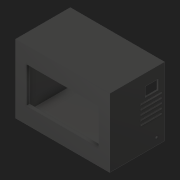
# Autodesk Inventor part: GA06
Saved by Autodesk Inventor 2017 (Build 210142000, 142)
## iProperties
Created: 2018-11-17
Part Number: GA06
Material: ABS Plastic
Document SubType Name: Modeling
Designer: Dell
Density: 1.06 g/cm^3
Appearance: Smooth - Black
Author: Dell
Autodesk Inventor part; units mm, degrees
ref_plane "YZ Plane" through (0, 0, 0) normal (1, 0, 0) x (0, 1, 0)
ref_plane "XZ Plane" through (0, 0, 0) normal (0, 1, 0) x (-1, 0, 0)
ref_plane "XY Plane" through (0, 0, 0) normal (0, 0, 1) x (1, 0, 0)
sketch "Sketch1" plane through (0, 0, 0) normal (0, 0, 1) x (1, 0, 0)
  line L0 (0, 0) -> (0, 70) construction
  circle A0 centre (0, 0) radius 2.5
  circle A1 centre (0, 70) radius 2.5
  line L1 (0, 0) -> (125, 0) construction
  circle A2 centre (125, 0) radius 2.5
  circle A3 centre (125, 70) radius 2.5
  line L2 (-8.5, -16) -> (133.5, -16)
  line L3 (133.5, -16) -> (133.5, 86)
  line L4 (133.5, 86) -> (-8.5, 86)
  line L5 (-8.5, 86) -> (-8.5, -16)
  point P0 (62.5, 0)
  point P1 (62.5, -16)
  point P2 (0, 35)
  point P3 (-8.5, 35)
  dimension "d0" = 70
  dimension "d1" = 5
  dimension "d2" = 5
  dimension "d3" = 5
  dimension "d4" = 5
  dimension "d5" = 125
  dimension "d6" = 142
  dimension "d7" = 102
  constraints: 12 end point, 4 centre point, 4 midpoint, 3 coincident, 2 horizontal, 2 horizontal alignment, 2 parallel, 2 vertical alignment, 1 perpendicular, 1 vertical
  measures "d0" distance of L0.start L0.end
  measures "d1" diameter of A0
  measures "d2" diameter of A1
  measures "d3" diameter of A2
  measures "d4" diameter of A3
  measures "d5" distance of L1.start L1.end
  measures "d6" distance of L4.end L3.end
  measures "d7" distance of L3.end L2.end
extrude "Extrusion1" add sketch "Sketch1" along normal blind 5
sketch "Sketch2" plane through (0, 0, 5) normal (0, 0, 1) x (1, 0, 0)
  line L0 (6.5, 60) -> (118.5, 60)
  line L1 (118.5, 60) -> (118.5, 10)
  line L2 (118.5, 10) -> (6.5, 10)
  line L3 (6.5, 10) -> (6.5, 60)
  line L4 (-8.5, 86) -> (-8.5, -16) projected
  line L5 (133.5, 86) -> (-8.5, 86) projected
  point P0 (0, 0)
  point P1 (62.5, 60)
  point P2 (62.5, 86)
  point P3 (6.5, 35)
  point P4 (-8.5, 35)
  dimension "d10" = 15
  dimension "d11" = 50
  constraints: 8 end point, 4 midpoint, 2 parallel, 1 horizontal, 1 horizontal alignment, 1 perpendicular, 1 vertical alignment
  measures "d10" distance between parallel lines of L4 L3
  measures "d11" distance of L0.end L1.end
extrude "Extrusion2" cut sketch "Sketch2" against normal through all
sketch "Sketch3" plane through (-8.5, 86, 0) normal (0, 1, 0) x (1, 0, 0)
  line L0 (142, 0) -> (142, -5) projected
  line L1 (142, -5) -> (0, -5)
  line L2 (0, -5) -> (0, 80)
  line L3 (0, 80) -> (142, 80)
  line L4 (142, 80) -> (142, -5)
  point P0 (8.5, 0)
  dimension "d17" = 85
  constraints: 8 end point, 2 parallel, 1 coincident, 1 horizontal, 1 perpendicular
  measures "d17" distance of L1.end L2.end
extrude "Extrusion3" add sketch "Sketch3" along normal blind 2
sketch "Sketch4" plane through (-8.5, -16, 0) normal (0, -1, 0) x (1, 0, 0)
  line L0 (142, 0) -> (0, 0) projected
  line L1 (0, 0) -> (0, -80) projected
  line L2 (0, -80) -> (142, -80) projected
  line L3 (142, -80) -> (142, 0) projected
  line L4 (0, 0) -> (142, 0) projected
  line L5 (142, 0) -> (142, 5) projected
  line L6 (0, 5) -> (142, 5) projected
  line L7 (0, 0) -> (0, 5) projected
  point P0 (8.5, 0)
extrude "Extrusion4" add sketch "Sketch4" along normal blind 2
sketch "Sketch5" plane through (-8.5, 86, -80) normal (-1, 0, 0) x (0, 0, 1)
  line L0 (85, -104) -> (85, 2) projected
  line L1 (0, -102) -> (0, -104) projected
  line L2 (85, 2) -> (0, 2)
  line L3 (0, 2) -> (0, -104)
  line L4 (0, -104) -> (85, -104)
  line L5 (85, -104) -> (85, 2)
  point P0 (80, -86)
  constraints: 8 end point, 2 parallel, 1 horizontal, 1 perpendicular
extrude "Extrusion5" add sketch "Sketch5" along normal blind 2
sketch "Sketch6" plane through (133.5, 86, 0) normal (1, 0, 0) x (0, 0, -1)
  line L0 (-5, -104) -> (-5, 2) projected
  line L1 (-5, -104) -> (80, -104)
  line L2 (80, -104) -> (80, 2)
  line L3 (80, 2) -> (-5, 2)
  line L4 (-5, 2) -> (-5, -104)
  point P0 (0, -86)
  constraints: 8 end point, 2 parallel, 1 horizontal, 1 perpendicular
extrude "Extrusion6" add sketch "Sketch6" along normal blind 2
sketch "Sketch7" plane through (0, 0, 5) normal (0, 0, 1) x (1, 0, 0)
  line L0 (118.5, 10) -> (6.5, 10) construction
  line L1 (6.5, 60) -> (118.5, 60) construction
  line L2 (6.5, 10) -> (6.5, 60) construction
  line L3 (118.5, 60) -> (118.5, 10) construction
  line L4 (6.5, 60) -> (61.5, 60)
  line L5 (61.5, 60) -> (61.5, 50)
  line L6 (61.5, 50) -> (6.5, 50)
  line L7 (6.5, 50) -> (6.5, 60)
  line L8 (118.5, 10) -> (63.5, 10)
  line L9 (63.5, 10) -> (63.5, 20)
  line L10 (63.5, 20) -> (118.5, 20)
  line L11 (118.5, 20) -> (118.5, 10)
  line L12 (118.5, 10) -> (6.5, 10) projected
  line L13 (6.5, 60) -> (118.5, 60) projected
  line L14 (6.5, 10) -> (6.5, 60) projected
  point P0 (0, 0)
  point P1 (62.5, 10)
  point P2 (62.5, 60)
  point P3 (6.5, 35)
  dimension "d26" = 55
  dimension "d27" = 10
  dimension "d28" = 55
  dimension "d29" = 10
  constraints: 24 end point, 6 midpoint, 4 parallel, 2 horizontal, 2 perpendicular
  measures "d26" distance of L5.end L6.end
  measures "d27" distance of L4.end L5.end
  measures "d28" distance of L9.end L10.end
  measures "d29" distance of L8.end L9.end
extrude "Extrusion7" add sketch "Sketch7" against normal blind 5
chamfer "Chamfer2" distance 3 angle 45 4 edges at (35, 10, 0) (90, 60, 0) (91, 20, 5) (34, 50, 5)
sketch "Sketch8" plane through (135.5, 86, 0) normal (1, 0, 0) x (0, 0, -1)
  line L0 (80, -104) -> (80, 2) projected
  line L1 (80, -102) -> (80, 0) projected
  line L2 (80, -51) -> (93.9386, -51)
  line L3 (80, -78.0836) -> (55, -78.0836)
  line L4 (55, -78.0836) -> (55, -58.0836)
  line L5 (55, -58.0836) -> (80, -58.0836)
  line L6 (80, -58.0836) -> (80, -78.0836)
  point P0 (0, -86)
  dimension "d36" = 20
  dimension "d37" = 25
  dimension "d40" = 7.0836
  constraints: 10 end point, 2 horizontal, 2 parallel, 1 midpoint, 1 perpendicular, 1 point on line
  measures "d36" distance between parallel lines of L5 L3
  measures "d37" distance of L4.end L5.end
  measures "d40" distance between parallel lines of L2 L5
extrude "Extrusion8" cut sketch "Sketch8" against normal blind 10
sketch "Sketch9" plane through (-10.5, 86, -80) normal (-1, 0, 0) x (0, 0, 1)
  line L0 (0, -58.0836) -> (0, 0) projected
  line L1 (0, -31) -> (25, -31)
  line L2 (25, -31) -> (25, -71)
  line L3 (25, -71) -> (0, -71)
  line L4 (0, -71) -> (0, -31)
  line L5 (0, 2) -> (0, -104) projected
  line L6 (0, -71) -> (25, -71)
  line L7 (25, -71) -> (25, -31)
  line L8 (25, -31) -> (0, -31)
  line L9 (0, -31) -> (0, -71)
  point P0 (80, -86)
  point P1 (0, -51)
  dimension "d41" = 40
  dimension "d42" = 25
  constraints: 16 end point, 4 parallel, 2 horizontal, 2 midpoint, 2 perpendicular, 1 point on line
  measures "d41" distance of L1.end L2.end
  measures "d42" distance of L1.start L1.end
extrude "Extrusion9" cut sketch "Sketch9" against normal blind 10
sketch "Sketch10" plane through (-10.5, 86, -80) normal (-1, 0, 0) x (0, 0, 1)
  circle A0 centre (12.5, -93) radius 1.5
  circle A1 centre (12.5, -9) radius 1.5
  line L0 (12.5, -93) -> (12.5, -9) construction
  line L1 (85, -104) -> (85, 2) projected
  line L2 (25, -71) -> (0, -71) projected
  point P0 (80, -86)
  point P1 (85, -51)
  point P2 (12.5, -51)
  point P3 (12.5, -71)
  point P4 (12.5, -71)
  dimension "d45" = 3
  dimension "d46" = 3
  dimension "d47" = 84
  constraints: 4 midpoint, 2 centre point, 2 end point, 1 horizontal alignment, 1 vertical, 1 vertical alignment
  measures "d45" diameter of A0
  measures "d46" diameter of A1
  measures "d47" distance of L0.start L0.end
extrude "Extrusion10" cut sketch "Sketch10" against normal blind 10
sketch "Sketch11" plane through (0, 0, 5) normal (0, 0, 1) x (1, 0, 0)
  circle A0 centre (0, 0) radius 2.5 projected
  circle A1 centre (0, 70) radius 2.5 projected
  circle A2 centre (125, 0) radius 2.5 projected
  circle A3 centre (125, 70) radius 2.5 projected
extrude "Extrusion11" add sketch "Sketch11" against normal blind 5
sketch "Sketch12" plane through (0, 0, 5) normal (0, 0, 1) x (1, 0, 0)
  line L0 (118.5, 20) -> (118.5, 63) projected
  line L1 (6.5, 7) -> (118.5, 7)
  line L2 (118.5, 7) -> (118.5, 63)
  line L3 (118.5, 63) -> (6.5, 63)
  line L4 (6.5, 63) -> (6.5, 7)
  point P0 (0, 0)
  constraints: 8 end point, 2 parallel, 1 coincident, 1 horizontal, 1 perpendicular
extrude "Extrusion12" cut sketch "Sketch12" along normal through all both and the other way through all
sketch "Sketch13" plane through (135.5, 86, 0) normal (1, 0, 0) x (0, 0, -1)
  line L0 (55, -58.0836) -> (80, -58.0836) projected
  line L1 (55, -78.0836) -> (55, -58.0836) projected
  line L2 (80, -78.0836) -> (55, -78.0836) projected
  line L3 (80, -58.0836) -> (80, -78.0836)
  line L4 (80, -71) -> (80, -102) projected
  point P0 (0, -86)
  constraints: 2 end point, 1 collinear
extrude "Extrusion13" add sketch "Sketch13" against normal blind 2
sketch "Sketch15" plane through (135.5, 86, 0) normal (1, 0, 0) x (0, 0, -1)
  line L0 (50, -31) -> (70, -31)
  line L1 (70, -31) -> (70, -16)
  line L2 (70, -16) -> (50, -16)
  line L3 (50, -16) -> (50, -31)
  line L4 (80, -104) -> (80, 2) projected
  line L5 (80, 2) -> (-5, 2) projected
  point P0 (0, -86)
  dimension "d64" = 20
  dimension "d65" = 15
  dimension "d66" = 10
  dimension "d67" = 18
  constraints: 8 end point, 2 parallel, 1 horizontal, 1 perpendicular
  measures "d64" distance of L2.end L1.end
  measures "d65" distance of L1.end L0.end
  measures "d66" distance between parallel lines of L4 L1
  measures "d67" distance between parallel lines of L5 L2
extrude "Extrusion15" cut sketch "Sketch15" against normal blind 10
sketch "Sketch16" plane through (135.5, 86, 0) normal (1, 0, 0) x (0, 0, -1)
  line L0 (70, -31) -> (50, -31) construction
  line L1 (50, -16) -> (70, -16) construction
  line L2 (50, -31) -> (50, -16) construction
  line L3 (70, -16) -> (70, -31) construction
  line L4 (70, -31) -> (70, -16) construction
  line L5 (70, -31) -> (38, -31) construction
  line L6 (38, -31) -> (38, -71) construction
  line L7 (38, -71) -> (80, -71) construction
  line L8 (80, -71) -> (80, -31) construction
  line L9 (43, -66) -> (43, -36) construction
  line L10 (43, -36) -> (75, -36) construction
  line L11 (75, -36) -> (75, -66) construction
  line L12 (75, -66) -> (43, -66) construction
  line L13 (43, -36) -> (75, -36)
  line L14 (75, -36) -> (75, -38)
  line L15 (75, -38) -> (43, -38)
  line L16 (43, -38) -> (43, -36)
  line L17 (75, -66) -> (43, -66)
  line L18 (43, -66) -> (43, -64)
  line L19 (43, -64) -> (75, -64)
  line L20 (75, -64) -> (75, -66)
  line L21 (75, -45) -> (43, -45)
  line L22 (43, -43) -> (75, -43) construction
  line L23 (43, -43) -> (75, -43)
  line L24 (75, -43) -> (75, -45)
  line L25 (43, -45) -> (43, -43)
  line L26 (75, -43) -> (75, -73) construction
  line L27 (75, -52) -> (43, -52)
  line L28 (43, -50) -> (75, -50) construction
  line L29 (43, -50) -> (75, -50)
  line L30 (75, -50) -> (75, -52)
  line L31 (43, -52) -> (43, -50)
  line L32 (75, -50) -> (75, -80) construction
  line L33 (75, -59) -> (43, -59)
  line L34 (43, -57) -> (75, -57) construction
  line L35 (43, -57) -> (75, -57)
  line L36 (75, -57) -> (75, -59)
  line L37 (43, -59) -> (43, -57)
  line L38 (75, -57) -> (75, -87) construction
  line L39 (75, -66) -> (43, -66)
  line L40 (43, -64) -> (75, -64) construction
  line L41 (43, -64) -> (75, -64)
  line L42 (75, -64) -> (75, -66)
  line L43 (43, -66) -> (43, -64)
  line L44 (75, -64) -> (75, -94) construction
  line L45 (80, -104) -> (80, 2) projected
  point P0 (0, -86)
  dimension "d70" = 42
  dimension "d71" = 40
  dimension "d72" = 5
  dimension "d73" = 2
  dimension "d74" = 2
  dimension "d77" = 7
  constraints: 80 end point, 8 parallel, 7 point on line, 4 perpendicular, 3 horizontal, 1 vertical, 51 other
  measures "d70" distance of L7.end L6.end
  measures "d71" distance of L6.end L5.end
  measures "d72" distance between parallel lines of L6 L9
  measures "d73" distance between parallel lines of L10 L15
  measures "d74" distance between parallel lines of L12 L19
  measures "d77" distance of L9.end L22.start
extrude "Extrusion16" cut sketch "Sketch16" against normal blind 10
sketch "Sketch17" plane through (135.5, 86, 0) normal (1, 0, 0) x (0, 0, -1)
  circle A0 centre (67.5, -93) radius 1.5 projected
  point P0 (0, -86)
extrude "Extrusion17" cut sketch "Sketch17" against normal blind 10
body "Solid1"
